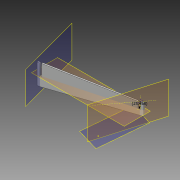
# Autodesk Inventor part: brace
Saved by Autodesk Inventor 2017 (Build 210142000, 142)
## iProperties
Created: 2018-10-17
Part Number: brace
Material: Generic
Document SubType Name: Modeling
Designer: ari
Density: 1 g/cm^3
Appearance: Default
Author: ari
Autodesk Inventor part; units mm, degrees
ref_plane "YZ Plane" through (0, 0, 0) normal (1, 0, 0) x (0, 1, 0)
ref_plane "XZ Plane" through (0, 0, 0) normal (0, 1, 0) x (-1, 0, 0)
sketch "Sketch1" plane through (0, 0, 0) normal (0, 0, 1) x (1, 0, 0)
  line L0 (-63.5719, 111.8382) -> (-7.6155, -96.5129) construction
  line L1 (-12.4444, -97.8098) -> (-68.7777, 111.945) construction
  line L2 (-42.0741, -26.0387) -> (-40.7772, -30.8676)
  line L3 (-40.7772, -30.8676) -> (304.995, 61.9956)
  line L4 (304.995, 61.9956) -> (303.6981, 66.8245)
  line L5 (-23.1781, -38.5663) -> (-40.7772, -30.8676) construction
  line L6 (247.1858, -96.9584) -> (307.8088, 111.597) construction
  line L7 (-42.0741, -26.0387) -> (-32.4163, -23.445) construction
  line L8 (294.0403, 64.2307) -> (303.6981, 66.8245) construction
  line L9 (-42.0741, -26.0387) -> (303.6981, 66.8245)
  point P0 (0, 0)
extrude "Extrusion1" add sketch "Sketch1" along normal blind 100
ref_plane "Work Plane1" through (0, 0, 50) normal (0, 0, 1) x (1, 0, 0)
sketch "Sketch3" plane through (0, 0, 100) normal (0, 0, 1) x (1, 0, 0)
  line L0 (302.6018, 111.597) -> (307.8088, 111.597) construction
  line L1 (302.6018, 111.597) -> (242.3845, -95.5627) construction
  line L2 (242.3845, -95.5627) -> (247.1858, -96.9584) construction
  line L3 (247.1858, -96.9584) -> (307.8088, 111.597) construction
  line L4 (-42.0741, -26.0387) -> (-40.7772, -30.8676) construction
  line L5 (-40.7772, -30.8676) -> (304.995, 61.9956) construction
  line L6 (304.995, 61.9956) -> (303.6981, 66.8245) construction
  line L7 (303.6981, 66.8245) -> (-42.0741, -26.0387) construction
  line L8 (285.4632, 61.9272) -> (286.7601, 57.0983)
  line L9 (286.7601, 57.0983) -> (295.3372, 59.4019)
  line L10 (295.3372, 59.4019) -> (294.0403, 64.2307)
  line L11 (294.0403, 64.2307) -> (285.4632, 61.9272)
  point P0 (0, 0)
  constraints: 8 end point, 5 point on line, 2 parallel, 1 perpendicular
extrude "Extrusion2" cut sketch "Sketch3" against normal up to surface (50 mm away)
sketch "Sketch4" plane through (0, 0, 100) normal (0, 0, 1) x (1, 0, 0)
  line L0 (286.7601, 57.0983) -> (285.4632, 61.9272) construction
  line L1 (285.4632, 61.9272) -> (-42.0741, -26.0387) construction
  line L2 (-42.0741, -26.0387) -> (-40.7772, -30.8676) construction
  line L3 (-40.7772, -30.8676) -> (286.7601, 57.0983) construction
  line L4 (-63.5719, 111.8382) -> (-68.7777, 111.945) construction
  line L5 (-12.4444, -97.8098) -> (-68.7777, 111.945) construction
  line L6 (-7.6155, -96.5129) -> (-12.4444, -97.8098) construction
  line L7 (-63.5719, 111.8382) -> (-7.6155, -96.5129) construction
  line L8 (-40.7772, -30.8676) -> (286.7601, 57.0983) construction
  line L9 (-32.4163, -23.445) -> (-31.1195, -28.2739)
  line L10 (-31.1195, -28.2739) -> (-26.2906, -26.977)
  line L11 (-26.2906, -26.977) -> (-27.5875, -22.1481)
  line L12 (-27.5875, -22.1481) -> (-32.4163, -23.445)
  line L13 (-32.6578, -23.5098) -> (-31.3609, -28.3387)
  line L14 (-31.3609, -28.3387) -> (-26.0491, -26.9121)
  line L15 (-26.0491, -26.9121) -> (-27.346, -22.0832)
  line L16 (-27.346, -22.0832) -> (-32.6578, -23.5098)
  line L17 (285.4632, 61.9272) -> (-42.0741, -26.0387) projected
  point P0 (0, 0)
  point P1 (-28.705, -27.6254)
  dimension "d21" = 5.5
  constraints: 16 end point, 6 point on line, 4 parallel, 2 midpoint, 2 perpendicular, 1 collinear
  measures "d21" distance of L13.end L14.end
extrude "Extrusion3" cut sketch "Sketch4" against normal up to surface (50 mm away)
ref_plane "Work Plane2" through (315.6821, 138.6828, 40.9) normal (0.0484699, 0.1667464, -0.9848078) x (-0.9602541, 0.2791272, 0)
ref_plane "Work Plane3" through (238.7196, -108.8102, 126.4793) normal (0, 0, -1) x (0, 1, 0)
sketch "Sketch6" plane through (303.6981, 66.8245, 100) normal (-0.2593763, 0.9657763, 0) x (0.9657763, 0.2593763, 0)
  line L0 (-348.2751, 50) -> (-342.7751, 50) construction
  line L1 (-18.881, 0) -> (-342.7751, 0) construction
  line L2 (-18.881, 0) -> (-18.881, 50) construction
  line L3 (-18.881, 50) -> (-10, 50) construction
  line L4 (-10, 50) -> (-10, 0) construction
  line L5 (0, 0) -> (-10, 0) construction
  line L6 (0, 100) -> (0, 0) construction
  line L7 (0, 100) -> (-358.0251, 100) construction
  line L8 (-358.0251, 100) -> (-358.0251, 0) construction
  line L9 (-14.0857, 72.7069) -> (0, 72.7069)
  line L10 (0, 100) -> (0, 0) construction
  line L11 (0, 72.7069) -> (0, 100)
  line L12 (-358.0251, 100) -> (0, 100) projected
  line L13 (0, 100) -> (-358.0251, 100)
  line L14 (-358.0251, 100) -> (-358.0251, 88.8925)
  line L15 (-358.0251, 100) -> (-358.0251, 0) construction
  line L16 (-343.0251, 88.8925) -> (-358.0251, 88.8925)
  line L17 (-343.0251, 88.8925) -> (-14.0857, 72.7069)
  line L18 (-358.0251, 100) -> (-358.0251, 0) construction
  line L19 (-342.7751, 50) -> (-342.7751, 0) projected
  line L20 (-348.2751, 0) -> (-358.0251, 0) projected
  line L21 (-348.2751, 0) -> (-348.2751, 50) projected
  point P0 (-310.6371, 100)
  constraints: 12 end point, 2 collinear, 2 perpendicular, 2 point on line, 2 other
extrude "Extrusion5" cut sketch "Sketch6" against normal through all
sketch "Sketch7" plane through (285.4632, 61.9272, 100) normal (-0.2593763, 0.9657763, 0) x (0.9657763, 0.2593763, 0)
  line L0 (18.881, 72.7069) -> (18.881, 0) construction
  line L1 (-339.1441, 88.8925) -> (-339.1441, 0) construction
  line L2 (-323.8941, 4.5) -> (-339.1441, 4.5)
  line L3 (-339.1441, 4.5) -> (-339.1441, 0)
  line L4 (-339.1441, 0) -> (18.881, 0) projected
  line L5 (-339.1441, 0) -> (18.881, 0)
  line L6 (8.881, 0) -> (18.881, 0) projected
  line L7 (18.881, 0) -> (18.881, 25)
  line L8 (0, 0) -> (0, 50) construction
  line L9 (18.881, 25) -> (0, 25)
  line L10 (0, 25) -> (-323.8941, 4.5)
  line L11 (0, 50) -> (8.881, 50) construction
  line L12 (-323.8941, 50) -> (-323.8941, 0) construction
  point P0 (-291.7561, 100)
  dimension "d17" = 25
  dimension "d18" = 4.5
  constraints: 12 end point, 3 point on line, 2 perpendicular, 1 midpoint
  measures "d17" distance from line of L7.end L11
  measures "d18" distance between parallel lines of L5 L2
ref_plane "Work Plane4" through (315.6821, 138.6828, 45.9) normal (0.9602541, -0.2791272, 0) x (0.2791272, 0.9602541, 0)
sketch "Sketch8" plane through (315.6821, 138.6828, 45.9) normal (0.9602541, -0.2791272, 0) x (0.2791272, 0.9602541, 0)
  line L0 (-245.3946, 71.5637) -> (-28.2069, 15.6815) construction
  line L1 (-82.1398, 54.1) -> (-82.1398, 4.1) construction
  point P0 (-221.2862, -45.9)
  point P1 (-82.1398, 29.5584)
  dimension "d16" = 25.4584
  constraints: 2 point on line
  measures "d16" distance of L1.end point (-82.14, 29.558)
ref_plane "Work Plane5" through (-76.0939, 139.1865, 45.8) normal (-0.9657763, -0.2593763, 0) x (-0.2593763, 0.9657763, 0)
extrude "Extrusion6" cut sketch "Sketch7" against normal through all
body "Solid1"
